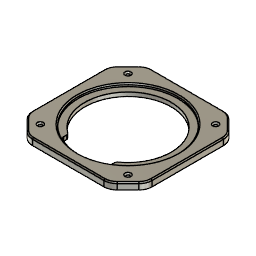
nextion_2.1inch_CNCed_enclosure (Autodesk Fusion 360 design; units mm, degrees)
Autodesk Fusion 360 part; units mm, degrees
note: some values were not read from the file. Set by a fixed rule: which sketch regions a step uses; the direction of a hole.
sketch "Sketch1" plane through (0, 0, 0) normal (0, 0, 1) x (1, 0, 0)
  circle A0 centre (0, 0) radius 37.5
  circle A1 centre (0, 0) radius 32.5
  circle A2 centre (0, 0) radius 36.5
  line L0 (-18, 0) -> (18, 0)
  line L1 (18, 0) -> (18, -31.753)
  line L2 (-18, 0) -> (-18, -31.753)
  line L3 (45, -45) -> (-45, -45)
  line L4 (-45, -45) -> (-45, 45)
  line L5 (-45, 45) -> (45, 45)
  line L6 (45, 45) -> (45, -45)
  line L7 (45, -45) -> (-45, 45) construction
  line L8 (-45, -45) -> (45, 45) construction
  dimension "d1" = 75
  dimension "d2" = -5
  dimension "d3" = -1
  dimension "d4" = 36
  dimension "d5" = 90
  dimension "d6" = 90
  constraint coincident A0.centre A1.centre
  constraint horizontal L0
  constraint midpoint A0.centre L0
  constraint coincident A2 L1.end
  constraint perpendicular L0 L1
  constraint coincident A2 L2.end
  constraint perpendicular L0 L2
  constraint horizontal L3
  constraint perpendicular L3 L4
  constraint parallel L3 L5
  constraint parallel L4 L6
  constraint coincident L7 A0.centre
  constraint coincident L8 A0.centre
  measures "d1" diameter of A0
  measures "d4" distance of L0.start L0.end
  measures "d5" distance of L4.end L5.end
  measures "d6" distance of L3.end L4.end
extrude "Extrude1" add sketch "Sketch1" along normal blind 5 contours L3 L4 L5 L6
extrude "Extrude2" add sketch "Sketch1" along normal blind 3 contours A0 | A1 A2 L1 L2 picked at (-19.5132, -29.1741)
chamfer "Chamfer1" distance 14 angle 45 4 edges at (-45, 45, 2.5) (45, 45, 2.5) (45, -45, 2.5) (-45, -45, 2.5)
fillet "Fillet1" radius 10 8 edges at (-31, 45, 2.5) (-45, 31, 2.5) (31, 45, 2.5) (45, 31, 2.5) (45, -31, 2.5) (31, -45, 2.5) (-31, -45, 2.5) (-45, -31, 2.5)
sketch "Sketch2" plane through (0, 0, 0) normal (0, 0, 1) x (1, 0, 0)
  line L0 (33, -33) -> (-33, -33)
  line L1 (-33, -33) -> (-33, 33)
  line L2 (-33, 33) -> (33, 33)
  line L3 (33, 33) -> (33, -33)
  line L4 (33, -33) -> (-33, 33) construction
  line L5 (-33, -33) -> (33, 33) construction
  dimension "d14" = 66
  dimension "d15" = 66
  constraint horizontal L0
  constraint perpendicular L0 L1
  constraint parallel L0 L2
  constraint parallel L1 L3
  constraint coincident L4 origin
  constraint coincident L5 origin
  measures "d14" distance of L1.end L2.end
  measures "d15" distance of L0.end L1.end
hole "Hole1" at (33, 33, 0) at (33, -33, 0) at (-33, -33, 0) at (-33, 33, 0) direction (0, 0, 1) diameter 2.5 depth 5 tip angle 180
chamfer "Chamfer2" distance 0.8 angle 45 16 edges at (0, 45, 5) (-30.6847, 44.2388, 5) (-38, 38, 5) (-44.2388, 30.6847, 5) (-45, 0, 5) (-44.2388, -30.6847, 5) (-38, -38, 5) (-30.6847, -44.2388, 5) (0, -45, 5) (30.6847, -44.2388, 5) (38, -38, 5) (44.2388, -30.6847, 5) (45, 0, 5) (44.2388, 30.6847, 5) (38, 38, 5) (30.6847, 44.2388, 5)
chamfer "Chamfer2" distance 0.8 angle 45 1 edges at (-34.9623, 13.5606, 5)
chamfer "Chamfer2" distance 1 angle 45 4 edges at (34.1654, 32.548, 5) (34.1654, -33.452, 5) (-31.8346, -33.452, 5) (-31.8346, 32.548, 5)
fillet "Fillet2" radius 2 4 edges at (-18, -31.753, 1.5) (-18, -27.0601, 1.5) (18, -31.753, 1.5) (18, -27.0601, 1.5)
named bodies: "nextion_2.1inch_CNCed_enclosure"
